Autodesk Inventor part; units mm, degrees
(part 5 of 10)
  spline S8 degree 5 poles (-8.528, -1.9637) (-8.5222, -1.9613) (-8.5144, -1.9581) (-8.5048, -1.9541) (-8.4933, -1.9493) (-8.4799, -1.9436) (-8.4704, -1.9395) (-8.461, -1.9354) (-8.4515, -1.9313) (-8.4421, -1.9272) (-8.4327, -1.9231) (-8.4234, -1.9189) (-8.4141, -1.9148) (-8.4048, -1.9106) (-8.3956, -1.9064) (-8.3864, -1.9022) (-8.3772, -1.898) (-8.3681, -1.8938) (-8.359, -1.8896) (-8.35, -1.8854) (-8.341, -1.8811) (-8.332, -1.8768) (-8.323, -1.8726) (-8.3141, -1.8683) (-8.3052, -1.864) (-8.2964, -1.8597) (-8.2876, -1.8553) (-8.2788, -1.851) (-8.2701, -1.8467) (-8.2614, -1.8423) (-8.251, -1.8371) (-8.2406, -1.8318) (-8.2303, -1.8266) (-8.2184, -1.8204) (-8.2065, -1.8142) (-8.1964, -1.8089) (-8.1864, -1.8036) (-8.1764, -1.7983) (-8.1664, -1.7929) (-8.1565, -1.7875) (-8.1467, -1.7822) (-8.1353, -1.7759) (-8.1239, -1.7696) (-8.1142, -1.7642) (-8.103, -1.7579) (-8.0919, -1.7515) (-8.0824, -1.7461) (-8.0714, -1.7397) (-8.0605, -1.7334) (-8.0512, -1.7279) (-8.0389, -1.7206) (-8.0266, -1.7133) (-8.016, -1.7069) (-8.0055, -1.7005) (-7.992, -1.6922) (-7.9817, -1.6858) (-7.9714, -1.6793) (-7.9612, -1.6729) (-7.9481, -1.6645) (-7.9381, -1.6581) (-7.9281, -1.6516) (-7.9168, -1.6442) (-7.9056, -1.6368) (-7.8973, -1.6312) (-7.8877, -1.6248) (-7.8781, -1.6183) (-7.8699, -1.6127) (-7.8605, -1.6062) (-7.8512, -1.5997) (-7.8432, -1.5942) (-7.834, -1.5877) (-7.8249, -1.5812) (-7.8171, -1.5756) (-7.8082, -1.5692) (-7.7993, -1.5627) (-7.7917, -1.5571) (-7.7829, -1.5507) (-7.7743, -1.5442) (-7.7669, -1.5387) (-7.7584, -1.5322) (-7.7499, -1.5258) (-7.7427, -1.5203) (-7.7344, -1.5138) (-7.7262, -1.5074) (-7.7192, -1.5019) (-7.7112, -1.4955) (-7.7032, -1.4891) (-7.6964, -1.4837) (-7.6885, -1.4773) (-7.6808, -1.4709) (-7.6742, -1.4655) (-7.6666, -1.4592) (-7.6591, -1.4529) (-7.6527, -1.4475) (-7.6453, -1.4412) (-7.638, -1.4349) (-7.6318, -1.4296) (-7.6247, -1.4234) (-7.6176, -1.4172) (-7.6116, -1.4119) (-7.6047, -1.4057) (-7.5979, -1.3995) (-7.5921, -1.3943) (-7.5854, -1.3882) (-7.5788, -1.3821) (-7.5732, -1.3769) (-7.5668, -1.3709) (-7.5604, -1.3649) (-7.555, -1.3598) (-7.5488, -1.3538) (-7.5427, -1.3479) (-7.5375, -1.3429) (-7.5315, -1.337) (-7.5256, -1.3312) (-7.5207, -1.3262) (-7.5149, -1.3204) (-7.5093, -1.3147) (-7.5045, -1.3098) (-7.499, -1.3041) (-7.4936, -1.2985) (-7.489, -1.2937) (-7.4837, -1.2882) (-7.4786, -1.2827) (-7.4742, -1.278) (-7.4692, -1.2725) (-7.4642, -1.2671) (-7.4601, -1.2625) (-7.4553, -1.2572) (-7.4506, -1.252) (-7.4466, -1.2475) (-7.4421, -1.2423) (-7.4376, -1.2372) (-7.4339, -1.2328) (-7.4296, -1.2278) (-7.4253, -1.2228) (-7.4218, -1.2186) (-7.4177, -1.2137) (-7.4137, -1.2089) (-7.4104, -1.2048) (-7.4065, -1.2001) (-7.4028, -1.1954) (-7.3996, -1.1915) (-7.3961, -1.1869) (-7.3925, -1.1824) (-7.3896, -1.1786) (-7.3862, -1.1743) (-7.383, -1.17) (-7.3802, -1.1664) (-7.3771, -1.1622) (-7.3741, -1.1581) (-7.3715, -1.1546) (-7.3686, -1.1507) (-7.3658, -1.1468) (-7.3635, -1.1435) (-7.3612, -1.1403) (-7.3583, -1.1361) (-7.3558, -1.1325) (-7.353, -1.1285) (-7.3504, -1.1246) (-7.3479, -1.1209) (-7.3461, -1.1181) (-7.3443, -1.1154) (-7.3429, -1.1132) (-7.3415, -1.1111) (-7.3402, -1.109) (-7.3388, -1.1069) (-7.3376, -1.1049) (-7.3364, -1.103) (-7.3352, -1.1011) (-7.334, -1.0992) (-7.3329, -1.0974) (-7.3319, -1.0957) (-7.3309, -1.094) (-7.3299, -1.0924) (-7.3289, -1.0908) (-7.328, -1.0892) (-7.3272, -1.0878) (-7.3264, -1.0864) (-7.3256, -1.085) (-7.3248, -1.0837) (-7.3241, -1.0824) (-7.3235, -1.0813) (-7.3229, -1.0801) (-7.3223, -1.0791) (-7.3217, -1.0781) (-7.3212, -1.0771) (-7.3208, -1.0763) (-7.3203, -1.0755) (-7.3199, -1.0747) (-7.3196, -1.074) (-7.3193, -1.0734) (-7.3189, -1.0728) (-7.3187, -1.0723) (-7.3186, -1.072) (-7.3185, -1.0718) (-7.3184, -1.0717) knots -1 -1 -1 -1 -1 -1 -0.9875 -0.983333 -0.979167 -0.975 -0.970833 -0.966667 -0.9625 -0.958333 -0.954167 -0.95 -0.945833 -0.941667 -0.9375 -0.933333 -0.929167 -0.925 -0.920833 -0.916667 -0.9125 -0.908333 -0.904167 -0.9 -0.895833 -0.891667 -0.8875 -0.883333 -0.879167 -0.875 -0.870833 -0.8625 -0.858333 -0.854167 -0.845833 -0.841667 -0.8375 -0.833333 -0.829167 -0.820833 -0.816667 -0.8125 -0.804167 -0.8 -0.795833 -0.7875 -0.783333 -0.779167 -0.770833 -0.766667 -0.7625 -0.75 -0.745833 -0.741667 -0.7375 -0.725 -0.720833 -0.716667 -0.7125 -0.7 -0.695833 -0.691667 -0.683333 -0.679167 -0.675 -0.666667 -0.6625 -0.658333 -0.65 -0.645833 -0.641667 -0.633333 -0.629167 -0.625 -0.616667 -0.6125 -0.608333 -0.6 -0.595833 -0.591667 -0.583333 -0.579167 -0.575 -0.566667 -0.5625 -0.558333 -0.55 -0.545833 -0.541667 -0.533333 -0.529167 -0.525 -0.516667 -0.5125 -0.508333 -0.5 -0.495833 -0.491667 -0.483333 -0.479167 -0.475 -0.466667 -0.4625 -0.458333 -0.45 -0.445833 -0.441667 -0.433333 -0.429167 -0.425 -0.416667 -0.4125 -0.408333 -0.4 -0.395833 -0.391667 -0.383333 -0.379167 -0.375 -0.366667 -0.3625 -0.358333 -0.35 -0.345833 -0.341667 -0.333333 -0.329167 -0.325 -0.316667 -0.3125 -0.308333 -0.3 -0.295833 -0.291667 -0.283333 -0.279167 -0.275 -0.266667 -0.2625 -0.258333 -0.25 -0.245833 -0.241667 -0.233333 -0.229167 -0.225 -0.216667 -0.2125 -0.208333 -0.2 -0.195833 -0.191667 -0.183333 -0.179167 -0.175 -0.170833 -0.158333 -0.154167 -0.145833 -0.141667 -0.1375 -0.133333 -0.129167 -0.125 -0.120833 -0.116667 -0.1125 -0.108333 -0.104167 -0.1 -0.095833 -0.091667 -0.0875 -0.083333 -0.079167 -0.075 -0.070833 -0.066667 -0.0625 -0.058333 -0.054167 -0.05 -0.045833 -0.041667 -0.0375 -0.033333 -0.029167 -0.025 -0.020833 -0.016667 -0.0125 -0.008333 0 0 0 0 0 0
  line L18 (-0.374, 5.4756) -> (0.4714, 5.7477)
  line L19 (0.4714, 5.7477) -> (0.472, 5.7479)
  spline S9 degree 5 poles (0.472, 5.7479) (0.4721, 5.7479) (0.4722, 5.748) (0.4724, 5.7481) (0.4728, 5.7482) (0.4733, 5.7483) (0.4738, 5.7485) (0.4745, 5.7488) (0.4752, 5.749) (0.476, 5.7493) (0.4768, 5.7496) (0.4778, 5.75) (0.4788, 5.7504) (0.4798, 5.7508) (0.4809, 5.7512) (0.4821, 5.7517) (0.4834, 5.7522) (0.4847, 5.7527) (0.4861, 5.7533) (0.4876, 5.7539) (0.4891, 5.7545) (0.4907, 5.7551) (0.4923, 5.7558) (0.494, 5.7566) (0.4957, 5.7573) (0.4976, 5.7581) (0.4994, 5.7589) (0.5014, 5.7598) (0.5033, 5.7607) (0.5054, 5.7616) (0.5075, 5.7625) (0.5096, 5.7635) (0.5123, 5.7647) (0.515, 5.766) (0.5178, 5.7674) (0.5212, 5.769) (0.5246, 5.7707) (0.5277, 5.7722) (0.5313, 5.774) (0.535, 5.7758) (0.5383, 5.7775) (0.5422, 5.7795) (0.5462, 5.7816) (0.5497, 5.7834) (0.5539, 5.7856) (0.5581, 5.7879) (0.5618, 5.79) (0.5662, 5.7924) (0.5707, 5.7949) (0.5746, 5.797) (0.5793, 5.7997) (0.584, 5.8024) (0.5881, 5.8047) (0.5929, 5.8076) (0.5979, 5.8105) (0.6022, 5.813) (0.6072, 5.8161) (0.6124, 5.8192) (0.6168, 5.8219) (0.6221, 5.8252) (0.6274, 5.8285) (0.632, 5.8314) (0.6375, 5.8349) (0.643, 5.8385) (0.6478, 5.8416) (0.6534, 5.8453) (0.6591, 5.849) (0.664, 5.8523) (0.6698, 5.8562) (0.6757, 5.8602) (0.6807, 5.8637) (0.6867, 5.8678) (0.6927, 5.872) (0.6979, 5.8757) (0.704, 5.88) (0.7102, 5.8844) (0.7155, 5.8883) (0.7218, 5.8929) (0.7281, 5.8975) (0.7335, 5.9015) (0.7399, 5.9063) (0.7464, 5.9112) (0.7519, 5.9154) (0.7585, 5.9204) (0.765, 5.9255) (0.7707, 5.93) (0.7774, 5.9352) (0.784, 5.9405) (0.7898, 5.9451) (0.7966, 5.9506) (0.8034, 5.9561) (0.8092, 5.9609) (0.8161, 5.9666) (0.823, 5.9723) (0.829, 5.9773) (0.8359, 5.9832) (0.8429, 5.9892) (0.849, 5.9944) (0.856, 6.0005) (0.8631, 6.0067) (0.8692, 6.0121) (0.8764, 6.0185) (0.8836, 6.0249) (0.8897, 6.0305) (0.897, 6.037) (0.9042, 6.0437) (0.9105, 6.0494) (0.9178, 6.0562) (0.9251, 6.0631) (0.9314, 6.0691) (0.9388, 6.0761) (0.9462, 6.0832) (0.9525, 6.0893) (0.96, 6.0966) (0.9674, 6.1039) (0.9738, 6.1102) (0.9813, 6.1177) (0.9888, 6.1252) (0.9953, 6.1318) (1.0028, 6.1395) (1.0104, 6.1472) (1.0169, 6.1539) (1.0244, 6.1618) (1.032, 6.1698) (1.0386, 6.1767) (1.0462, 6.1849) (1.0538, 6.1931) (1.0604, 6.2002) (1.0681, 6.2085) (1.0757, 6.217) (1.0823, 6.2243) (1.09, 6.2328) (1.0977, 6.2415) (1.1043, 6.249) (1.112, 6.2577) (1.1197, 6.2666) (1.1264, 6.2743) (1.1341, 6.2833) (1.1418, 6.2924) (1.1485, 6.3002) (1.1562, 6.3095) (1.164, 6.3188) (1.1706, 6.3268) (1.1784, 6.3362) (1.1861, 6.3458) (1.1928, 6.354) (1.2005, 6.3637) (1.2083, 6.3734) (1.215, 6.3818) (1.2216, 6.3903) (1.2316, 6.4031) (1.2404, 6.4145) (1.2493, 6.4261) (1.2582, 6.4378) (1.2692, 6.4525) (1.277, 6.4629) (1.2847, 6.4734) (1.2924, 6.484) (1.3035, 6.4992) (1.3123, 6.5114) (1.3211, 6.5238) (1.3299, 6.5362) (1.3387, 6.5488) (1.3442, 6.5567) (1.3496, 6.5647) (1.3551, 6.5726) (1.3606, 6.5806) (1.3661, 6.5887) (1.3715, 6.5968) (1.377, 6.6049) (1.3824, 6.613) (1.3879, 6.6212) (1.3933, 6.6295) (1.3987, 6.6377) (1.4041, 6.646) (1.4096, 6.6544) (1.415, 6.6628) (1.4204, 6.6712) (1.4258, 6.6796) (1.4312, 6.6881) (1.4365, 6.6966) (1.4419, 6.7052) (1.4473, 6.7138) (1.4526, 6.7224) (1.458, 6.7311) (1.4633, 6.7398) (1.4687, 6.7486) (1.474, 6.7573) (1.4793, 6.7662) (1.4846, 6.775) (1.4899, 6.7839) (1.4973, 6.7964) (1.5036, 6.8071) (1.5089, 6.8162) (1.5131, 6.8234) (1.5162, 6.8289) knots 0 0 0 0 0 0 0.004167 0.008333 0.0125 0.016667 0.020833 0.025 0.029167 0.033333 0.0375 0.041667 0.045833 0.05 0.054167 0.058333 0.0625 0.066667 0.070833 0.075 0.079167 0.083333 0.0875 0.091667 0.095833 0.1 0.104167 0.108333 0.1125 0.116667 0.120833 0.125 0.129167 0.1375 0.141667 0.145833 0.154167 0.158333 0.1625 0.170833 0.175 0.179167 0.1875 0.191667 0.195833 0.204167 0.208333 0.2125 0.220833 0.225 0.229167 0.2375 0.241667 0.245833 0.254167 0.258333 0.2625 0.270833 0.275 0.279167 0.2875 0.291667 0.295833 0.304167 0.308333 0.3125 0.320833 0.325 0.329167 0.3375 0.341667 0.345833 0.354167 0.358333 0.3625 0.370833 0.375 0.379167 0.3875 0.391667 0.395833 0.404167 0.408333 0.4125 0.420833 0.425 0.429167 0.4375 0.441667 0.445833 0.454167 0.458333 0.4625 0.470833 0.475 0.479167 0.4875 0.491667 0.495833 0.504167 0.508333 0.5125 0.520833 0.525 0.529167 0.5375 0.541667 0.545833 0.554167 0.558333 0.5625 0.570833 0.575 0.579167 0.5875 0.591667 0.595833 0.604167 0.608333 0.6125 0.620833 0.625 0.629167 0.6375 0.641667 0.645833 0.654167 0.658333 0.6625 0.670833 0.675 0.679167 0.6875 0.691667 0.695833 0.704167 0.708333 0.7125 0.720833 0.725 0.729167 0.7375 0.741667 0.745833 0.754167 0.758333 0.7625 0.770833 0.775 0.779167 0.783333 0.8 0.804167 0.808333 0.8125 0.825 0.829167 0.833333 0.8375 0.854167 0.858333 0.8625 0.866667 0.870833 0.875 0.879167 0.883333 0.8875 0.891667 0.895833 0.9 0.904167 0.908333 0.9125 0.916667 0.920833 0.925 0.929167 0.933333 0.9375 0.941667 0.945833 0.95 0.954167 0.958333 0.9625 0.966667 0.970833 0.975 0.979167 0.983333 0.9875 1 1 1 1 1 1
  arc A10 (1.5162, 6.8289) -> (1.2422, 7.3858) centre (-4.8955, 4.02) ccw
  spline S10 degree 5 poles (1.2422, 7.3858) (1.236, 7.3866) (1.2277, 7.3877) (1.2173, 7.3891) (1.2049, 7.3906) (1.1905, 7.3924) (1.1802, 7.3936) (1.17, 7.3948) (1.1598, 7.396) (1.1496, 7.3971) (1.1394, 7.3982) (1.1292, 7.3993) (1.1191, 7.4003) (1.109, 7.4014) (1.0989, 7.4024) (1.0888, 7.4033) (1.0788, 7.4043) (1.0688, 7.4052) (1.0588, 7.4061) (1.0488, 7.4069) (1.0389, 7.4077) (1.029, 7.4085) (1.0191, 7.4093) (1.0092, 7.4101) (0.9994, 7.4108) (0.9896, 7.4115) (0.9798, 7.4121) (0.97, 7.4128) (0.9603, 7.4134) (0.9506, 7.4139) (0.939, 7.4146) (0.9274, 7.4152) (0.9158, 7.4158) (0.9024, 7.4164) (0.8891, 7.417) (0.8776, 7.4175) (0.8663, 7.4179) (0.8549, 7.4183) (0.8436, 7.4186) (0.8324, 7.4189) (0.8212, 7.4192) (0.8082, 7.4195) (0.7952, 7.4197) (0.7841, 7.4199) (0.7712, 7.42) (0.7584, 7.4201) (0.7475, 7.4201) (0.7348, 7.4201) (0.7221, 7.42) (0.7114, 7.42) (0.697, 7.4198) (0.6828, 7.4196) (0.6704, 7.4193) (0.658, 7.419) (0.6423, 7.4186) (0.6301, 7.4182) (0.6179, 7.4178) (0.6059, 7.4173) (0.5904, 7.4166) (0.5785, 7.416) (0.5666, 7.4154) (0.5548, 7.4147) (0.5397, 7.4138) (0.5281, 7.4131) (0.5165, 7.4123) (0.5033, 7.4113) (0.4903, 7.4103) (0.4805, 7.4095) (0.4692, 7.4085) (0.458, 7.4075) (0.4484, 7.4067) (0.4373, 7.4056) (0.4262, 7.4045) (0.4168, 7.4035) (0.4059, 7.4023) (0.395, 7.4011) (0.3858, 7.4001) (0.3751, 7.3988) (0.3645, 7.3975) (0.3554, 7.3963) (0.3449, 7.395) (0.3344, 7.3936) (0.3256, 7.3923) (0.3153, 7.3909) (0.305, 7.3894) (0.2963, 7.3881) (0.2863, 7.3865) (0.2763, 7.3849) (0.2677, 7.3836) (0.2579, 7.3819) (0.2481, 7.3803) (0.2398, 7.3788) (0.2301, 7.3771) (0.2206, 7.3754) (0.2124, 7.3739) (0.203, 7.3721) (0.1937, 7.3703) (0.1857, 7.3687) (0.1765, 7.3669) (0.1674, 7.365) (0.1597, 7.3634) (0.1507, 7.3614) (0.1419, 7.3595) (0.1343, 7.3578) (0.1256, 7.3559) (0.117, 7.3539) (0.1097, 7.3521) (0.1012, 7.3501) (0.0928, 7.3481) (0.0857, 7.3463) (0.0775, 7.3442) (0.0693, 7.3422) (0.0624, 7.3404) (0.0544, 7.3382) (0.0465, 7.3361) (0.0399, 7.3343) (0.0321, 7.3321) (0.0245, 7.33) (0.018, 7.3281) (0.0106, 7.326) (0.0032, 7.3238) (-0.003, 7.3219) (-0.0103, 7.3197) (-0.0174, 7.3175) (-0.0234, 7.3156) (-0.0303, 7.3134) (-0.0372, 7.3112) (-0.0429, 7.3093) (-0.0496, 7.3071) (-0.0562, 7.3049) (-0.0617, 7.303) (-0.0681, 7.3008) (-0.0744, 7.2986) (-0.0797, 7.2967) (-0.0858, 7.2945) (-0.0918, 7.2923) (-0.0969, 7.2904) (-0.1027, 7.2883) (-0.1084, 7.2861) (-0.1133, 7.2842) (-0.1188, 7.2821) (-0.1242, 7.2799) (-0.1288, 7.2781) (-0.134, 7.276) (-0.1392, 7.2739) (-0.1435, 7.2721) (-0.1484, 7.27) (-0.1532, 7.2679) (-0.1573, 7.2662) (-0.1619, 7.2642) (-0.1665, 7.2622) (-0.1702, 7.2605) (-0.1746, 7.2585) (-0.1788, 7.2566) (-0.1823, 7.255) (-0.1863, 7.2531) (-0.1902, 7.2512) (-0.1935, 7.2497) (-0.1972, 7.2479) (-0.2007, 7.2461) (-0.2037, 7.2447) (-0.2066, 7.2432) (-0.2094, 7.2418) (-0.2117, 7.2406) (-0.2139, 7.2395) (-0.216, 7.2384) (-0.2181, 7.2373) (-0.2202, 7.2362) (-0.2221, 7.2351) (-0.2241, 7.2341) (-0.2259, 7.2331) (-0.2277, 7.2321) (-0.2294, 7.2311) (-0.2311, 7.2302) (-0.2327, 7.2293) (-0.2342, 7.2284) (-0.2357, 7.2276) (-0.2371, 7.2268) (-0.2385, 7.226) (-0.2398, 7.2252) (-0.241, 7.2245) (-0.2422, 7.2238) (-0.2433, 7.2231) (-0.2443, 7.2225) (-0.2453, 7.2219) (-0.2462, 7.2214) (-0.247, 7.2208) (-0.2478, 7.2204) (-0.2485, 7.2199) (-0.2492, 7.2195) (-0.2497, 7.2191) (-0.2503, 7.2187) (-0.2508, 7.2185) (-0.2511, 7.2183) (-0.2512, 7.2182) (-0.2513, 7.2181) knots -1 -1 -1 -1 -1 -1 -0.9875 -0.983333 -0.979167 -0.975 -0.970833 -0.966667 -0.9625 -0.958333 -0.954167 -0.95 -0.945833 -0.941667 -0.9375 -0.933333 -0.929167 -0.925 -0.920833 -0.916667 -0.9125 -0.908333 -0.904167 -0.9 -0.895833 -0.891667 -0.8875 -0.883333 -0.879167 -0.875 -0.870833 -0.8625 -0.858333 -0.854167 -0.845833 -0.841667 -0.8375 -0.833333 -0.829167 -0.820833 -0.816667 -0.8125 -0.804167 -0.8 -0.795833 -0.7875 -0.783333 -0.779167 -0.770833 -0.766667 -0.7625 -0.75 -0.745833 -0.741667 -0.7375 -0.725 -0.720833 -0.716667 -0.7125 -0.7 -0.695833 -0.691667 -0.6875 -0.675 -0.670833 -0.666667 -0.658333 -0.654167 -0.65 -0.641667 -0.6375 -0.633333 -0.625 -0.620833 -0.616667 -0.608333 -0.604167 -0.6 -0.591667 -0.5875 -0.583333 -0.575 -0.570833 -0.566667 -0.558333 -0.554167 -0.55 -0.541667 -0.5375 -0.533333 -0.525 -0.520833 -0.516667 -0.508333 -0.504167 -0.5 -0.491667 -0.4875 -0.483333 -0.475 -0.470833 -0.466667 -0.458333 -0.454167 -0.45 -0.441667 -0.4375 -0.433333 -0.425 -0.420833 -0.416667 -0.408333 -0.404167 -0.4 -0.391667 -0.3875 -0.383333 -0.375 -0.370833 -0.366667 -0.358333 -0.354167 -0.35 -0.341667 -0.3375 -0.333333 -0.325 -0.320833 -0.316667 -0.308333 -0.304167 -0.3 -0.291667 -0.2875 -0.283333 -0.275 -0.270833 -0.266667 -0.258333 -0.254167 -0.25 -0.241667 -0.2375 -0.233333 -0.225 -0.220833 -0.216667 -0.208333 -0.204167 -0.2 -0.191667 -0.1875 -0.183333 -0.175 -0.170833 -0.166667 -0.158333 -0.154167 -0.15 -0.141667 -0.1375 -0.133333 -0.129167 -0.125 -0.120833 -0.116667 -0.1125 -0.108333 -0.104167 -0.1 -0.095833 -0.091667 -0.0875 -0.083333 -0.079167 -0.075 -0.070833 -0.066667 -0.0625 -0.058333 -0.054167 -0.05 -0.045833 -0.041667 -0.0375 -0.033333 -0.029167 -0.025 -0.020833 -0.016667 -0.0125 -0.008333 0 0 0 0 0 0
  line L20 (-0.2519, 7.2177) -> (-0.9834, 6.714)
  line L21 (-0.2513, 7.2181) -> (-0.2519, 7.2177)
  arc A11 (-0.9834, 6.714) -> (-1.7076, 7.5413) centre (-4.8955, 4.02) ccw
  line L22 (-1.7076, 7.5413) -> (-1.1115, 8.1997)
  line L23 (-2.4726, 9.1117) -> (-2.4729, 9.1111)
  line L24 (-2.4729, 9.1111) -> (-2.8545, 8.3091)
  spline S11 degree 5 poles (-1.1111, 8.2002) (-1.111, 8.2002) (-1.1109, 8.2003) (-1.1108, 8.2005) (-1.1105, 8.2008) (-1.1102, 8.2012) (-1.1098, 8.2016) (-1.1094, 8.2022) (-1.1089, 8.2027) (-1.1083, 8.2034) (-1.1078, 8.2041) (-1.1071, 8.2048) (-1.1065, 8.2057) (-1.1057, 8.2066) (-1.105, 8.2075) (-1.1042, 8.2085) (-1.1033, 8.2096) (-1.1024, 8.2107) (-1.1015, 8.2119) (-1.1006, 8.2131) (-1.0996, 8.2144) (-1.0985, 8.2158) (-1.0975, 8.2172) (-1.0964, 8.2186) (-1.0952, 8.2202) (-1.094, 8.2218) (-1.0928, 8.2234) (-1.0916, 8.2251) (-1.0903, 8.2269) (-1.089, 8.2287) (-1.0877, 8.2306) (-1.0863, 8.2325) (-1.0846, 8.2349) (-1.0829, 8.2373) (-1.0811, 8.2399) (-1.079, 8.243) (-1.0769, 8.2462) (-1.075, 8.249) (-1.0727, 8.2524) (-1.0704, 8.2559) (-1.0684, 8.259) (-1.0664, 8.2621) (-1.064, 8.2659) (-1.0608, 8.2709) (-1.0576, 8.2761) (-1.0543, 8.2815) (-1.0509, 8.287) (-1.0475, 8.2928) (-1.0448, 8.2973) (-1.0421, 8.302) (-1.0393, 8.3067) (-1.0362, 8.3123) (-1.0333, 8.3173) (-1.0309, 8.3216) (-1.0281, 8.3268) (-1.0252, 8.3321) (-1.0227, 8.3367) (-1.0198, 8.3421) (-1.0168, 8.3477) (-1.0143, 8.3525) (-1.0113, 8.3582) (-1.0083, 8.3641) (-1.0057, 8.3692) (-1.0027, 8.3752) (-0.9996, 8.3813) (-0.997, 8.3866) (-0.9939, 8.3929) (-0.9908, 8.3992) (-0.9882, 8.4048) (-0.9851, 8.4113) (-0.982, 8.418) (-0.9793, 8.4238) (-0.9762, 8.4306) (-0.9731, 8.4375) (-0.9704, 8.4435) (-0.9672, 8.4506) (-0.9641, 8.4578) (-0.9614, 8.464) (-0.9582, 8.4713) (-0.9551, 8.4788) (-0.9524, 8.4852) (-0.9492, 8.4928) (-0.9461, 8.5005) (-0.9434, 8.5072) (-0.9403, 8.515) (-0.9371, 8.523) (-0.9344, 8.5298) (-0.9313, 8.5379) (-0.9282, 8.5461) (-0.9255, 8.5532) (-0.9224, 8.5616) (-0.9193, 8.57) (-0.9166, 8.5773) (-0.9136, 8.5859) (-0.9105, 8.5946) (-0.9079, 8.6021) (-0.9048, 8.6109) (-0.9018, 8.6199) (-0.8992, 8.6276) (-0.8961, 8.6366) (-0.8931, 8.6458) (-0.8906, 8.6537) (-0.8876, 8.663) (-0.8846, 8.6724) (-0.8821, 8.6805) (-0.8792, 8.6901) (-0.8763, 8.6997) (-0.8738, 8.708) (-0.8709, 8.7178) (-0.8681, 8.7276) (-0.8656, 8.7361) (-0.8628, 8.7461) (-0.86, 8.7562) (-0.8576, 8.7649) (-0.8549, 8.7751) (-0.8522, 8.7854) (-0.8498, 8.7942) (-0.8471, 8.8047) (-0.8445, 8.8152) (-0.8422, 8.8242) (-0.8396, 8.8349) (-0.837, 8.8456) (-0.8348, 8.8548) (-0.8323, 8.8657) (-0.8298, 8.8766) (-0.8276, 8.886) (-0.8252, 8.8971) (-0.8228, 8.9082) (-0.8207, 8.9178) (-0.8183, 8.9291) (-0.816, 8.9405) (-0.814, 8.9502) (-0.8117, 8.9617) (-0.8095, 8.9732) (-0.8076, 8.9832) (-0.8054, 8.9949) (-0.8032, 9.0066) (-0.8014, 9.0167) (-0.7993, 9.0286) (-0.7972, 9.0405) (-0.7955, 9.0508) (-0.7935, 9.0629) (-0.7915, 9.075) (-0.7899, 9.0854) (-0.788, 9.0977) (-0.7862, 9.11) (-0.7846, 9.1206) (-0.7826, 9.1348) (-0.7806, 9.1491) (-0.7789, 9.1617) (-0.7772, 9.1743) (-0.7756, 9.1871) (-0.7738, 9.2017) (-0.7721, 9.2163) (-0.7704, 9.2311) (-0.7688, 9.2459) (-0.767, 9.2628) (-0.7659, 9.274) (-0.7648, 9.2853) (-0.7633, 9.3004) (-0.762, 9.3156) (-0.7608, 9.329) (-0.7597, 9.3424) (-0.7586, 9.3559) (-0.7579, 9.3656) (-0.7572, 9.3753) (-0.7565, 9.3851) (-0.7558, 9.3948) (-0.7552, 9.4046) (-0.7546, 9.4144) (-0.754, 9.4243) (-0.7534, 9.4341) (-0.7529, 9.444) (-0.7524, 9.454) (-0.7519, 9.4639) (-0.7514, 9.4739) (-0.7509, 9.4839) (-0.7505, 9.494) (-0.7501, 9.5041) (-0.7498, 9.5142) (-0.7494, 9.5243) (-0.7491, 9.5344) (-0.7488, 9.5446) (-0.7485, 9.5548) (-0.7483, 9.5651) (-0.748, 9.5753) (-0.7479, 9.5856) (-0.7477, 9.5959) (-0.7475, 9.6063) (-0.7474, 9.6208) (-0.7473, 9.6333) (-0.7472, 9.6437) (-0.7472, 9.6521) (-0.7472, 9.6584) knots 0 0 0 0 0 0 0.004167 0.008333 0.0125 0.016667 0.020833 0.025 0.029167 0.033333 0.0375 0.041667 0.045833 0.05 0.054167 0.058333 0.0625 0.066667 0.070833 0.075 0.079167 0.083333 0.0875 0.091667 0.095833 0.1 0.104167 0.108333 0.1125 0.116667 0.120833 0.125 0.129167 0.1375 0.141667 0.145833 0.154167 0.158333 0.1625 0.170833 0.175 0.179167 0.183333 0.191667 0.208333 0.2125 0.216667 0.220833 0.229167 0.2375 0.241667 0.245833 0.254167 0.258333 0.2625 0.270833 0.275 0.279167 0.2875 0.291667 0.295833 0.304167 0.308333 0.3125 0.320833 0.325 0.329167 0.3375 0.341667 0.345833 0.354167 0.358333 0.3625 0.370833 0.375 0.379167 0.3875 0.391667 0.395833 0.404167 0.408333 0.4125 0.420833 0.425 0.429167 0.4375 0.441667 0.445833 0.454167 0.458333 0.4625 0.470833 0.475 0.479167 0.4875 0.491667 0.495833 0.504167 0.508333 0.5125 0.520833 0.525 0.529167 0.5375 0.541667 0.545833 0.554167 0.558333 0.5625 0.570833 0.575 0.579167 0.5875 0.591667 0.595833 0.604167 0.608333 0.6125 0.620833 0.625 0.629167 0.6375 0.641667 0.645833 0.654167 0.658333 0.6625 0.670833 0.675 0.679167 0.6875 0.691667 0.695833 0.704167 0.708333 0.7125 0.720833 0.725 0.729167 0.7375 0.741667 0.745833 0.754167 0.758333 0.7625 0.770833 0.775 0.779167 0.791667 0.795833 0.8 0.804167 0.808333 0.825 0.829167 0.833333 0.8375 0.845833 0.85 0.854167 0.866667 0.870833 0.875 0.879167 0.883333 0.8875 0.891667 0.895833 0.9 0.904167 0.908333 0.9125 0.916667 0.920833 0.925 0.929167 0.933333 0.9375 0.941667 0.945833 0.95 0.954167 0.958333 0.9625 0.966667 0.970833 0.975 0.979167 0.983333 0.9875 1 1 1 1 1 1
  arc A12 (-0.7472, 9.6584) -> (-1.263, 10.0037) centre (-4.8955, 4.02) ccw
  spline S12 degree 5 poles (-1.263, 10.0037) (-1.2688, 10.0013) (-1.2766, 9.9981) (-1.2862, 9.9941) (-1.2977, 9.9892) (-1.3111, 9.9836) (-1.3206, 9.9795) (-1.33, 9.9754) (-1.3395, 9.9713) (-1.3489, 9.9672) (-1.3583, 9.963) (-1.3676, 9.9589) (-1.3769, 9.9548) (-1.3862, 9.9506) (-1.3954, 9.9464) (-1.4046, 9.9422) (-1.4138, 9.938) (-1.4229, 9.9338) (-1.432, 9.9296) (-1.441, 9.9253) (-1.45, 9.9211) (-1.459, 9.9168) (-1.468, 9.9125) (-1.4769, 9.9082) (-1.4858, 9.9039) (-1.4946, 9.8996) (-1.5034, 9.8953) (-1.5122, 9.891) (-1.5209, 9.8866) (-1.5296, 9.8823) (-1.54, 9.877) (-1.5504, 9.8718) (-1.5607, 9.8665) (-1.5726, 9.8604) (-1.5844, 9.8542) (-1.5946, 9.8489) (-1.6046, 9.8436) (-1.6146, 9.8382) (-1.6246, 9.8329) (-1.6345, 9.8275) (-1.6443, 9.8221) (-1.6557, 9.8159) (-1.6671, 9.8096) (-1.6768, 9.8042) (-1.688, 9.7978) (-1.6991, 9.7915) (-1.7086, 9.7861) (-1.7196, 9.7797) (-1.7305, 9.7733) (-1.7398, 9.7679) (-1.7521, 9.7606) (-1.7644, 9.7533) (-1.775, 9.7468) (-1.7855, 9.7404) (-1.799, 9.7322) (-1.8093, 9.7257) (-1.8196, 9.7193) (-1.8298, 9.7128) (-1.8429, 9.7045) (-1.8529, 9.698) (-1.8629, 9.6916) (-1.8742, 9.6842) (-1.8854, 9.6768) (-1.8937, 9.6712) (-1.9033, 9.6647) (-1.9129, 9.6582) (-1.9211, 9.6527) (-1.9305, 9.6462) (-1.9398, 9.6397) (-1.9478, 9.6341) (-1.957, 9.6277) (-1.9661, 9.6212) (-1.9739, 9.6156) (-1.9828, 9.6091) (-1.9917, 9.6027) (-1.9993, 9.5971) (-2.0081, 9.5906) (-2.0167, 9.5842) (-2.0241, 9.5786) (-2.0326, 9.5722) (-2.0411, 9.5657) (-2.0483, 9.5602) (-2.0566, 9.5538) (-2.0648, 9.5474) (-2.0718, 9.5419) (-2.0798, 9.5355) (-2.0878, 9.5291) (-2.0946, 9.5236) (-2.1025, 9.5173) (-2.1102, 9.5109) (-2.1168, 9.5055) (-2.1244, 9.4992) (-2.1319, 9.4928) (-2.1383, 9.4875) (-2.1457, 9.4812) (-2.153, 9.4749) (-2.1592, 9.4696) (-2.1663, 9.4633) (-2.1734, 9.4571) (-2.1794, 9.4518) (-2.1863, 9.4457) (-2.1931, 9.4395) (-2.1989, 9.4343) (-2.2056, 9.4282) (-2.2122, 9.4221) (-2.2178, 9.4169) (-2.2242, 9.4109) (-2.2306, 9.4049) (-2.236, 9.3998) (-2.2422, 9.3938) (-2.2483, 9.3879) (-2.2535, 9.3828) (-2.2595, 9.377) (-2.2654, 9.3711) (-2.2703, 9.3662) (-2.2761, 9.3604) (-2.2817, 9.3547) (-2.2865, 9.3498) (-2.292, 9.3441) (-2.2974, 9.3385) (-2.302, 9.3337) (-2.3073, 9.3281) (-2.3124, 9.3226) (-2.3168, 9.3179) (-2.3218, 9.3125) (-2.3268, 9.3071) (-2.3309, 9.3025) (-2.3357, 9.2972) (-2.3404, 9.2919) (-2.3444, 9.2874) (-2.3489, 9.2823) (-2.3534, 9.2771) (-2.3571, 9.2728) (-2.3614, 9.2677) (-2.3657, 9.2628) (-2.3692, 9.2585) (-2.3733, 9.2537) (-2.3773, 9.2488) (-2.3806, 9.2447) (-2.3845, 9.24) (-2.3882, 9.2354) (-2.3913, 9.2314) (-2.3949, 9.2269) (-2.3985, 9.2224) (-2.4014, 9.2186) (-2.4048, 9.2142) (-2.408, 9.2099) (-2.4108, 9.2063) (-2.4139, 9.2021) (-2.4169, 9.1981) (-2.4195, 9.1946) (-2.4224, 9.1906) (-2.4252, 9.1868) (-2.4275, 9.1835) (-2.4298, 9.1803) (-2.4327, 9.1761) (-2.4352, 9.1725) (-2.438, 9.1685) (-2.4406, 9.1646) (-2.4431, 9.1608) (-2.4449, 9.1581) (-2.4467, 9.1554) (-2.4481, 9.1532) (-2.4495, 9.1511) (-2.4508, 9.149) (-2.4522, 9.1469) (-2.4534, 9.1449) (-2.4546, 9.143) (-2.4558, 9.1411) (-2.457, 9.1392) (-2.4581, 9.1374) (-2.4591, 9.1357) (-2.4601, 9.134) (-2.4611, 9.1323) (-2.4621, 9.1307) (-2.463, 9.1292) (-2.4638, 9.1277) (-2.4646, 9.1263) (-2.4654, 9.125) (-2.4662, 9.1237) (-2.4669, 9.1224) (-2.4675, 9.1212) (-2.4681, 9.1201) (-2.4687, 9.119) (-2.4693, 9.118) (-2.4698, 9.1171) (-2.4702, 9.1162) (-2.4707, 9.1154) (-2.4711, 9.1147) (-2.4714, 9.114) (-2.4717, 9.1134) (-2.4721, 9.1128) (-2.4723, 9.1123) (-2.4724, 9.112) (-2.4725, 9.1118) (-2.4726, 9.1117) knots -1 -1 -1 -1 -1 -1 -0.9875 -0.983333 -0.979167 -0.975 -0.970833 -0.966667 -0.9625 -0.958333 -0.954167 -0.95 -0.945833 -0.941667 -0.9375 -0.933333 -0.929167 -0.925 -0.920833 -0.916667 -0.9125 -0.908333 -0.904167 -0.9 -0.895833 -0.891667 -0.8875 -0.883333 -0.879167 -0.875 -0.870833 -0.8625 -0.858333 -0.854167 -0.845833 -0.841667 -0.8375 -0.833333 -0.829167 -0.820833 -0.816667 -0.8125 -0.804167 -0.8 -0.795833 -0.7875 -0.783333 -0.779167 -0.770833 -0.766667 -0.7625 -0.75 -0.745833 -0.741667 -0.7375 -0.725 -0.720833 -0.716667 -0.7125 -0.7 -0.695833 -0.691667 -0.683333 -0.679167 -0.675 -0.666667 -0.6625 -0.658333 -0.65 -0.645833 -0.641667 -0.633333 -0.629167 -0.625 -0.616667 -0.6125 -0.608333 -0.6 -0.595833 -0.591667 -0.583333 -0.579167 -0.575 -0.566667 -0.5625 -0.558333 -0.55 -0.545833 -0.541667 -0.533333 -0.529167 -0.525 -0.516667 -0.5125 -0.508333 -0.5 -0.495833 -0.491667 -0.483333 -0.479167 -0.475 -0.466667 -0.4625 -0.458333 -0.45 -0.445833 -0.441667 -0.433333 -0.429167 -0.425 -0.416667 -0.4125 -0.408333 -0.4 -0.395833 -0.391667 -0.383333 -0.379167 -0.375 -0.366667 -0.3625 -0.358333 -0.35 -0.345833 -0.341667 -0.333333 -0.329167 -0.325 -0.316667 -0.3125 -0.308333 -0.3 -0.295833 -0.291667 -0.283333 -0.279167 -0.275 -0.266667 -0.2625 -0.258333 -0.25 -0.245833 -0.241667 -0.233333 -0.229167 -0.225 -0.216667 -0.2125 -0.208333 -0.2 -0.195833 -0.191667 -0.183333 -0.179167 -0.175 -0.170833 -0.158333 -0.154167 -0.145833 -0.141667 -0.1375 -0.133333 -0.129167 -0.125 -0.120833 -0.116667 -0.1125 -0.108333 -0.104167 -0.1 -0.095833 -0.091667 -0.0875 -0.083333 -0.079167 -0.075 -0.070833 -0.066667 -0.0625 -0.058333 -0.054167 -0.05 -0.045833 -0.041667 -0.0375 -0.033333 -0.029167 -0.025 -0.020833 -0.016667 -0.0125 -0.008333 0 0 0 0 0 0
  line L25 (-1.1115, 8.1997) -> (-1.1111, 8.2002)
  arc A13 (-2.8545, 8.3091) -> (-3.8953, 8.6635) centre (-4.8955, 4.02) ccw
  line L26 (-3.7083, 9.5317) -> (-3.7082, 9.5324)
  line L27 (-3.8953, 8.6635) -> (-3.7083, 9.5317)
  spline S13 degree 5 poles (-3.7082, 9.5324) (-3.7082, 9.5324) (-3.7081, 9.5326) (-3.7081, 9.5328) (-3.708, 9.5331) (-3.7079, 9.5336) (-3.7078, 9.5342) (-3.7077, 9.5349) (-3.7076, 9.5357) (-3.7074, 9.5365) (-3.7073, 9.5374) (-3.7071, 9.5384) (-3.7069, 9.5394) (-3.7068, 9.5405) (-3.7066, 9.5417) (-3.7064, 9.543) (-3.7062, 9.5443) (-3.706, 9.5458) (-3.7058, 9.5472) (-3.7056, 9.5488) (-3.7053, 9.5504) (-3.7051, 9.5521) (-3.7049, 9.5539) (-3.7047, 9.5557) (-3.7044, 9.5576) (-3.7042, 9.5596) (-3.704, 9.5616) (-3.7038, 9.5637) (-3.7035, 9.5659) (-3.7033, 9.5681) (-3.7031, 9.5704) (-3.7029, 9.5727) (-3.7026, 9.5756) (-3.7024, 9.5786) (-3.7021, 9.5817) (-3.7018, 9.5854) (-3.7016, 9.5893) (-3.7013, 9.5927) (-3.7011, 9.5967) (-3.7008, 9.6009) (-3.7006, 9.6046) (-3.7004, 9.609) (-3.7002, 9.6135) (-3.7001, 9.6174) (-3.6999, 9.6221) (-3.6998, 9.6269) (-3.6997, 9.6312) (-3.6996, 9.6362) (-3.6995, 9.6413) (-3.6994, 9.6458) (-3.6994, 9.6511) (-3.6993, 9.6566) (-3.6994, 9.6613) (-3.6994, 9.6669) (-3.6994, 9.6726) (-3.6995, 9.6776) (-3.6996, 9.6835) (-3.6997, 9.6895) (-3.6999, 9.6948) (-3.7001, 9.7009) (-3.7003, 9.7072) (-3.7005, 9.7127) (-3.7008, 9.7191) (-3.7011, 9.7257) (-3.7014, 9.7314) (-3.7018, 9.7381) (-3.7022, 9.7449) (-3.7026, 9.7508) (-3.7031, 9.7578) (-3.7036, 9.7649) (-3.7041, 9.771) (-3.7047, 9.7782) (-3.7053, 9.7855) (-3.7059, 9.7919) (-3.7066, 9.7993) (-3.7073, 9.8069) (-3.708, 9.8134) (-3.7088, 9.8211) (-3.7097, 9.8289) (-3.7105, 9.8357) (-3.7114, 9.8436) (-3.7124, 9.8516) (-3.7133, 9.8585) (-3.7144, 9.8667) (-3.7155, 9.8749) (-3.7165, 9.882) (-3.7177, 9.8904) (-3.7189, 9.8989) (-3.7201, 9.9062) (-3.7214, 9.9147) (-3.7228, 9.9234) (-3.724, 9.9309) (-3.7255, 9.9397) (-3.727, 9.9485) (-3.7284, 9.9562) (-3.73, 9.9652) (-3.7317, 9.9742) (-3.7332, 9.982) (-3.7349, 9.9912) (-3.7368, 10.0005) (-3.7384, 10.0084) (-3.7403, 10.0178) (-3.7423, 10.0272) (-3.744, 10.0354) (-3.7461, 10.0449) (-3.7482, 10.0545) (-3.7501, 10.0628) (-3.7523, 10.0725) (-3.7546, 10.0823) (-3.7566, 10.0908) (-3.759, 10.1007) (-3.7615, 10.1106) (-3.7636, 10.1192) (-3.7662, 10.1293) (-3.7688, 10.1394) (-3.7711, 10.1481) (-3.7738, 10.1583) (-3.7765, 10.1686) (-3.779, 10.1774) (-3.7819, 10.1878) (-3.7848, 10.1982) (-3.7874, 10.2072) (-3.7904, 10.2177) (-3.7936, 10.2283) (-3.7963, 10.2374) (-3.7995, 10.2481) (-3.8028, 10.2588) (-3.8057, 10.268) (-3.8091, 10.2789) (-3.8125, 10.2897) (-3.8155, 10.2991) (-3.8191, 10.31) (-3.8228, 10.321) (-3.8259, 10.3305) (-3.8297, 10.3415) (-3.8335, 10.3527) (-3.8368, 10.3622) (-3.8408, 10.3734) (-3.8448, 10.3847) (-3.8483, 10.3943) (-3.8524, 10.4057) (-3.8566, 10.417) (-3.8602, 10.4268) (-3.8645, 10.4382) (-3.8689, 10.4497) (-3.8727, 10.4596) (-3.8772, 10.4711) (-3.8817, 10.4827) (-3.8857, 10.4927) (-3.8897, 10.5027) (-3.8958, 10.5177) (-3.9013, 10.5311) (-3.9069, 10.5446) (-3.9125, 10.5581) (-3.9198, 10.5751) (-3.9249, 10.587) (-3.9301, 10.5989) (-3.9354, 10.6109) (-3.9423, 10.6263) (-3.9477, 10.6384) (-3.9532, 10.6504) (-3.9595, 10.6643) (-3.966, 10.6781) (-3.9709, 10.6886) (-3.9758, 10.699) (-3.9808, 10.7095) (-3.985, 10.7182) (-3.9893, 10.727) (-3.9936, 10.7358) (-3.9979, 10.7446) (-4.0022, 10.7533) (-4.0066, 10.7622) (-4.011, 10.771) (-4.0154, 10.7798) (-4.0199, 10.7887) (-4.0244, 10.7975) (-4.029, 10.8064) (-4.0336, 10.8153) (-4.0382, 10.8242) (-4.0428, 10.8331) (-4.0475, 10.842) (-4.0523, 10.851) (-4.057, 10.8599) (-4.0618, 10.8689) (-4.0667, 10.8778) (-4.0715, 10.8868) (-4.0764, 10.8958) (-4.0814, 10.9048) (-4.0864, 10.9138) (-4.0914, 10.9228) (-4.0964, 10.9318) (-4.1035, 10.9445) (-4.1097, 10.9554) (-4.1149, 10.9644) (-4.119, 10.9717) (-4.1222, 10.9771) knots 0 0 0 0 0 0 0.004167 0.008333 0.0125 0.016667 0.020833 0.025 0.029167 0.033333 0.0375 0.041667 0.045833 0.05 0.054167 0.058333 0.0625 0.066667 0.070833 0.075 0.079167 0.083333 0.0875 0.091667 0.095833 0.1 0.104167 0.108333 0.1125 0.116667 0.120833 0.125 0.129167 0.1375 0.141667 0.145833 0.154167 0.158333 0.1625 0.170833 0.175 0.179167 0.1875 0.191667 0.195833 0.204167 0.208333 0.2125 0.220833 0.225 0.229167 0.2375 0.241667 0.245833 0.254167 0.258333 0.2625 0.270833 0.275 0.279167 0.2875 0.291667 0.295833 0.304167 0.308333 0.3125 0.320833 0.325 0.329167 0.3375 0.341667 0.345833 0.354167 0.358333 0.3625 0.370833 0.375 0.379167 0.3875 0.391667 0.395833 0.404167 0.408333 0.4125 0.420833 0.425 0.429167 0.4375 0.441667 0.445833 0.454167 0.458333 0.4625 0.470833 0.475 0.479167 0.4875 0.491667 0.495833 0.504167 0.508333 0.5125 0.520833 0.525 0.529167 0.5375 0.541667 0.545833 0.554167 0.558333 0.5625 0.570833 0.575 0.579167 0.5875 0.591667 0.595833 0.604167 0.608333 0.6125 0.620833 0.625 0.629167 0.6375 0.641667 0.645833 0.654167 0.658333 0.6625 0.670833 0.675 0.679167 0.6875 0.691667 0.695833 0.704167 0.708333 0.7125 0.720833 0.725 0.729167 0.7375 0.741667 0.745833 0.754167 0.758333 0.7625 0.770833 0.775 0.779167 0.783333 0.8 0.804167 0.808333 0.8125 0.825 0.829167 0.833333 0.8375 0.85 0.854167 0.858333 0.866667 0.870833 0.875 0.879167 0.883333 0.8875 0.891667 0.895833 0.9 0.904167 0.908333 0.9125 0.916667 0.920833 0.925 0.929167 0.933333 0.9375 0.941667 0.945833 0.95 0.954167 0.958333 0.9625 0.966667 0.970833 0.975 0.979167 0.983333 0.9875 1 1 1 1 1 1
  line L28 (-5.343, 9.6404) -> (-5.2725, 8.755)
  line L29 (-5.3431, 9.641) -> (-5.343, 9.6404)
  arc A14 (-4.1222, 10.9771) -> (-4.7415, 11.0183) centre (-4.8955, 4.02) ccw
  arc A15 (-5.2725, 8.755) -> (-6.3511, 8.5415) centre (-4.8955, 4.02) ccw
  spline S14 degree 5 poles (-4.7415, 11.0183) (-4.7454, 11.0133) (-4.7505, 11.0067) (-4.7568, 10.9984) (-4.7643, 10.9884) (-4.7731, 10.9768) (-4.7793, 10.9685) (-4.7854, 10.9602) (-4.7916, 10.952) (-4.7976, 10.9437) (-4.8037, 10.9355) (-4.8097, 10.9272) (-4.8157, 10.9189) (-4.8216, 10.9107) (-4.8275, 10.9025) (-4.8334, 10.8942) (-4.8392, 10.886) (-4.845, 10.8778) (-4.8508, 10.8696) (-4.8565, 10.8614) (-4.8622, 10.8532) (-4.8678, 10.845) (-4.8735, 10.8368) (-4.879, 10.8287) (-4.8846, 10.8205) (-4.8901, 10.8123) (-4.8955, 10.8042) (-4.901, 10.7961) (-4.9064, 10.7879) (-4.9117, 10.7798) (-4.9181, 10.7701) (-4.9244, 10.7604) (-4.9307, 10.7507) (-4.938, 10.7394) (-4.9451, 10.7281) (-4.9513, 10.7184) (-4.9573, 10.7088) (-4.9633, 10.6992) (-4.9692, 10.6896) (-4.9751, 10.68) (-4.981, 10.6704) (-4.9877, 10.6592) (-4.9944, 10.6481) (-5.0001, 10.6386) (-5.0066, 10.6275) (-5.0131, 10.6165) (-5.0186, 10.607) (-5.0249, 10.596) (-5.0312, 10.585) (-5.0365, 10.5756) (-5.0427, 10.5647) (-5.0488, 10.5538) (-5.0539, 10.5445) (-5.0607, 10.5321) (-5.0674, 10.5198) (-5.0732, 10.509) (-5.0789, 10.4982) (-5.0862, 10.4845) (-5.0917, 10.4738) (-5.0972, 10.4632) (-5.1027, 10.4526) (-5.1095, 10.439) (-5.1148, 10.4285) (-5.12, 10.418) (-5.1259, 10.406) (-5.1316, 10.3942) (-5.1359, 10.3853) (-5.1408, 10.3749) (-5.1457, 10.3646) (-5.1498, 10.3558) (-5.1545, 10.3456) (-5.1592, 10.3354) (-5.1631, 10.3268) (-5.1676, 10.3167) (-5.1721, 10.3066) (-5.1759, 10.298) (-5.1802, 10.288) (-5.1845, 10.2781) (-5.1881, 10.2696) (-5.1923, 10.2598) (-5.1964, 10.25) (-5.1998, 10.2416) (-5.2038, 10.2319) (-5.2077, 10.2222) (-5.211, 10.214) (-5.2148, 10.2044) (-5.2185, 10.1949) (-5.2217, 10.1867) (-5.2253, 10.1773) (-5.2288, 10.1679) (-5.2318, 10.1599) (-5.2353, 10.1506) (-5.2386, 10.1414) (-5.2415, 10.1335) (-5.2447, 10.1244) (-5.2479, 10.1153) (-5.2506, 10.1076) (-5.2537, 10.0986) (-5.2567, 10.0897) (-5.2592, 10.0821) (-5.2621, 10.0734) (-5.265, 10.0646) (-5.2673, 10.0572) (-5.2701, 10.0486) (-5.2728, 10.04) (-5.275, 10.0327) (-5.2776, 10.0243) (-5.2801, 10.0159) (-5.2822, 10.0088) (-5.2846, 10.0005) (-5.2869, 9.9923) (-5.2889, 9.9853) (-5.2911, 9.9773) (-5.2933, 9.9693) (-5.2951, 9.9625) (-5.2972, 9.9546) (-5.2992, 9.9468) (-5.3009, 9.9402) (-5.3029, 9.9326) (-5.3047, 9.925) (-5.3063, 9.9185) (-5.3081, 9.9111) (-5.3098, 9.9037) (-5.3112, 9.8975) (-5.3129, 9.8903) (-5.3145, 9.8831) (-5.3158, 9.8771) (-5.3173, 9.8701) (-5.3187, 9.8632) (-5.3199, 9.8573) (-5.3212, 9.8505) (-5.3225, 9.8439) (-5.3236, 9.8382) (-5.3248, 9.8317) (-5.326, 9.8253) (-5.327, 9.8198) (-5.328, 9.8136) (-5.3291, 9.8074) (-5.3299, 9.8022) (-5.3309, 9.7962) (-5.3318, 9.7903) (-5.3326, 9.7853) (-5.3334, 9.7796) (-5.3342, 9.7739) (-5.3349, 9.7692) (-5.3356, 9.7637) (-5.3363, 9.7584) (-5.3368, 9.7538) (-5.3374, 9.7487) (-5.338, 9.7436) (-5.3385, 9.7394) (-5.339, 9.7345) (-5.3395, 9.7297) (-5.3399, 9.7257) (-5.3403, 9.7218) (-5.3407, 9.7167) (-5.3411, 9.7123) (-5.3414, 9.7075) (-5.3418, 9.7028) (-5.3421, 9.6983) (-5.3423, 9.695) (-5.3425, 9.6918) (-5.3426, 9.6892) (-5.3427, 9.6866) (-5.3429, 9.6841) (-5.343, 9.6817) (-5.3431, 9.6793) (-5.3431, 9.677) (-5.3432, 9.6748) (-5.3433, 9.6726) (-5.3433, 9.6705) (-5.3434, 9.6685) (-5.3434, 9.6665) (-5.3434, 9.6646) (-5.3435, 9.6628) (-5.3435, 9.661) (-5.3435, 9.6593) (-5.3435, 9.6576) (-5.3435, 9.6561) (-5.3435, 9.6546) (-5.3435, 9.6531) (-5.3434, 9.6518) (-5.3434, 9.6505) (-5.3434, 9.6493) (-5.3434, 9.6481) (-5.3433, 9.6471) (-5.3433, 9.6461) (-5.3433, 9.6452) (-5.3432, 9.6443) (-5.3432, 9.6436) (-5.3432, 9.6429) (-5.3431, 9.6422) (-5.3431, 9.6417) (-5.3431, 9.6413) (-5.3431, 9.6411) (-5.3431, 9.641) knots -1 -1 -1 -1 -1 -1 -0.9875 -0.983333 -0.979167 -0.975 -0.970833 -0.966667 -0.9625 -0.958333 -0.954167 -0.95 -0.945833 -0.941667 -0.9375 -0.933333 -0.929167 -0.925 -0.920833 -0.916667 -0.9125 -0.908333 -0.904167 -0.9 -0.895833 -0.891667 -0.8875 -0.883333 -0.879167 -0.875 -0.870833 -0.8625 -0.858333 -0.854167 -0.845833 -0.841667 -0.8375 -0.833333 -0.829167 -0.820833 -0.816667 -0.8125 -0.804167 -0.8 -0.795833 -0.7875 -0.783333 -0.779167 -0.770833 -0.766667 -0.7625 -0.754167 -0.75 -0.745833 -0.733333 -0.729167 -0.725 -0.720833 -0.708333 -0.704167 -0.7 -0.695833 -0.683333 -0.679167 -0.675 -0.666667 -0.6625 -0.658333 -0.65 -0.645833 -0.641667 -0.633333 -0.629167 -0.625 -0.616667 -0.6125 -0.608333 -0.6 -0.595833 -0.591667 -0.583333 -0.579167 -0.575 -0.566667 -0.5625 -0.558333 -0.55 -0.545833 -0.541667 -0.533333 -0.529167 -0.525 -0.516667 -0.5125 -0.508333 -0.5 -0.495833 -0.491667 -0.483333 -0.479167 -0.475 -0.466667 -0.4625 -0.458333 -0.45 -0.445833 -0.441667 -0.433333 -0.429167 -0.425 -0.416667 -0.4125 -0.408333 -0.4 -0.395833 -0.391667 -0.383333 -0.379167 -0.375 -0.366667 -0.3625 -0.358333 -0.35 -0.345833 -0.341667 -0.333333 -0.329167 -0.325 -0.316667 -0.3125 -0.308333 -0.3 -0.295833 -0.291667 -0.283333 -0.279167 -0.275 -0.266667 -0.2625 -0.258333 -0.25 -0.245833 -0.241667 -0.233333 -0.229167 -0.225 -0.216667 -0.2125 -0.208333 -0.2 -0.195833 -0.191667 -0.183333 -0.179167 -0.175 -0.170833 -0.158333 -0.154167 -0.145833 -0.141667 -0.1375 -0.133333 -0.129167 -0.125 -0.120833 -0.116667 -0.1125 -0.108333 -0.104167 -0.1 -0.095833 -0.091667 -0.0875 -0.083333 -0.079167 -0.075 -0.070833 -0.066667 -0.0625 -0.058333 -0.054167 -0.05 -0.045833 -0.041667 -0.0375 -0.033333 -0.029167 -0.025 -0.020833 -0.016667 -0.0125 -0.008333 0 0 0 0 0 0
  line L30 (-6.3511, 8.5415) -> (-6.6232, 9.3869)
  line L31 (-6.6232, 9.3869) -> (-6.6234, 9.3875)
  line L32 (-8.0932, 8.6636) -> (-7.5895, 7.9321)
  spline S15 degree 5 poles (-6.6234, 9.3875) (-6.6235, 9.3876) (-6.6235, 9.3877) (-6.6236, 9.3879) (-6.6237, 9.3882) (-6.6239, 9.3887) (-6.6241, 9.3893) (-6.6243, 9.39) (-6.6246, 9.3907) (-6.6248, 9.3915) (-6.6252, 9.3923) (-6.6255, 9.3932) (-6.6259, 9.3942) (-6.6263, 9.3953) (-6.6267, 9.3964) (-6.6272, 9.3976) (-6.6277, 9.3989) (-6.6282, 9.4002) (-6.6288, 9.4016) (-6.6294, 9.4031) (-6.63, 9.4046) (-6.6307, 9.4061) (-6.6314, 9.4078) (-6.6321, 9.4095) (-6.6328, 9.4112) (-6.6336, 9.413) (-6.6344, 9.4149) (-6.6353, 9.4168) (-6.6362, 9.4188) (-6.6371, 9.4209) (-6.638, 9.423) (-6.639, 9.4251) (-6.6403, 9.4278) (-6.6415, 9.4305) (-6.6429, 9.4333) (-6.6445, 9.4366) (-6.6462, 9.4401) (-6.6477, 9.4432) (-6.6495, 9.4468) (-6.6514, 9.4505) (-6.653, 9.4538) (-6.655, 9.4577) (-6.6571, 9.4617) (-6.659, 9.4652) (-6.6612, 9.4694) (-6.6635, 9.4736) (-6.6655, 9.4773) (-6.6679, 9.4817) (-6.6704, 9.4862) (-6.6726, 9.4901) (-6.6752, 9.4948) (-6.6779, 9.4995) (-6.6803, 9.5036) (-6.6831, 9.5084) (-6.686, 9.5134) (-6.6886, 9.5176) (-6.6916, 9.5227) (-6.6947, 9.5278) (-6.6975, 9.5323) (-6.7007, 9.5376) (-6.704, 9.5429) (-6.707, 9.5475) (-6.7104, 9.553) (-6.714, 9.5585) (-6.7171, 9.5632) (-6.7208, 9.5689) (-6.7245, 9.5746) (-6.7278, 9.5795) (-6.7317, 9.5853) (-6.7357, 9.5912) (-6.7392, 9.5962) (-6.7433, 9.6022) (-6.7475, 9.6082) (-6.7512, 9.6134) (-6.7555, 9.6195) (-6.76, 9.6257) (-6.7638, 9.631) (-6.7684, 9.6373) (-6.773, 9.6436) (-6.7771, 9.649) (-6.7818, 9.6554) (-6.7867, 9.6619) (-6.7909, 9.6674) (-6.796, 9.674) (-6.801, 9.6805) (-6.8055, 9.6862) (-6.8107, 9.6928) (-6.816, 9.6995) (-6.8206, 9.7053) (-6.8261, 9.7121) (-6.8316, 9.7189) (-6.8364, 9.7247) (-6.8421, 9.7316) (-6.8479, 9.7385) (-6.8528, 9.7444) (-6.8587, 9.7514) (-6.8647, 9.7584) (-6.8699, 9.7644) (-6.876, 9.7715) (-6.8822, 9.7786) (-6.8876, 9.7847) (-6.894, 9.7919) (-6.9004, 9.799) (-6.906, 9.8052) (-6.9125, 9.8124) (-6.9192, 9.8197) (-6.925, 9.8259) (-6.9318, 9.8332) (-6.9386, 9.8406) (-6.9446, 9.8469) (-6.9516, 9.8543) (-6.9587, 9.8616) (-6.9648, 9.868) (-6.9721, 9.8754) (-6.9794, 9.8829) (-6.9857, 9.8893) (-6.9932, 9.8968) (-7.0008, 9.9043) (-7.0073, 9.9108) (-7.015, 9.9183) (-7.0227, 9.9259) (-7.0295, 9.9323) (-7.0374, 9.9399) (-7.0454, 9.9475) (-7.0523, 9.9541) (-7.0604, 9.9617) (-7.0686, 9.9693) (-7.0757, 9.9759) (-7.0841, 9.9835) (-7.0925, 9.9912) (-7.0998, 9.9978) (-7.1083, 10.0055) (-7.117, 10.0132) (-7.1245, 10.0198) (-7.1333, 10.0275) (-7.1421, 10.0352) (-7.1498, 10.0418) (-7.1588, 10.0496) (-7.1679, 10.0573) (-7.1757, 10.064) (-7.185, 10.0717) (-7.1943, 10.0795) (-7.2023, 10.0861) (-7.2118, 10.0939) (-7.2213, 10.1016) (-7.2295, 10.1083) (-7.2392, 10.116) (-7.2489, 10.1238) (-7.2573, 10.1304) (-7.2658, 10.1371) (-7.2786, 10.1471) (-7.29, 10.1559) (-7.3016, 10.1648) (-7.3133, 10.1736) (-7.328, 10.1847) (-7.3384, 10.1925) (-7.3489, 10.2002) (-7.3595, 10.2079) (-7.3747, 10.219) (-7.3869, 10.2278) (-7.3993, 10.2366) (-7.4118, 10.2454) (-7.4243, 10.2542) (-7.4322, 10.2596) (-7.4402, 10.2651) (-7.4481, 10.2706) (-7.4562, 10.2761) (-7.4642, 10.2815) (-7.4723, 10.287) (-7.4804, 10.2924) (-7.4886, 10.2979) (-7.4968, 10.3033) (-7.505, 10.3088) (-7.5133, 10.3142) (-7.5216, 10.3196) (-7.5299, 10.325) (-7.5383, 10.3305) (-7.5467, 10.3359) (-7.5552, 10.3413) (-7.5636, 10.3466) (-7.5722, 10.352) (-7.5807, 10.3574) (-7.5893, 10.3628) (-7.598, 10.3681) (-7.6066, 10.3735) (-7.6153, 10.3788) (-7.6241, 10.3841) (-7.6329, 10.3895) (-7.6417, 10.3948) (-7.6505, 10.4001) (-7.6594, 10.4054) (-7.6719, 10.4128) (-7.6827, 10.4191) (-7.6917, 10.4244) (-7.6989, 10.4286) (-7.7044, 10.4317) knots 0 0 0 0 0 0 0.004167 0.008333 0.0125 0.016667 0.020833 0.025 0.029167 0.033333 0.0375 0.041667 0.045833 0.05 0.054167 0.058333 0.0625 0.066667 0.070833 0.075 0.079167 0.083333 0.0875 0.091667 0.095833 0.1 0.104167 0.108333 0.1125 0.116667 0.120833 0.125 0.129167 0.1375 0.141667 0.145833 0.154167 0.158333 0.1625 0.170833 0.175 0.179167 0.1875 0.191667 0.195833 0.204167 0.208333 0.2125 0.220833 0.225 0.229167 0.2375 0.241667 0.245833 0.254167 0.258333 0.2625 0.270833 0.275 0.279167 0.2875 0.291667 0.295833 0.304167 0.308333 0.3125 0.320833 0.325 0.329167 0.3375 0.341667 0.345833 0.354167 0.358333 0.3625 0.370833 0.375 0.379167 0.3875 0.391667 0.395833 0.404167 0.408333 0.4125 0.420833 0.425 0.429167 0.4375 0.441667 0.445833 0.454167 0.458333 0.4625 0.470833 0.475 0.479167 0.4875 0.491667 0.495833 0.504167 0.508333 0.5125 0.520833 0.525 0.529167 0.5375 0.541667 0.545833 0.554167 0.558333 0.5625 0.570833 0.575 0.579167 0.5875 0.591667 0.595833 0.604167 0.608333 0.6125 0.620833 0.625 0.629167 0.6375 0.641667 0.645833 0.654167 0.658333 0.6625 0.670833 0.675 0.679167 0.6875 0.691667 0.695833 0.704167 0.708333 0.7125 0.720833 0.725 0.729167 0.7375 0.741667 0.745833 0.754167 0.758333 0.7625 0.770833 0.775 0.779167 0.783333 0.8 0.804167 0.808333 0.8125 0.825 0.829167 0.833333 0.8375 0.854167 0.858333 0.8625 0.866667 0.870833 0.875 0.879167 0.883333 0.8875 0.891667 0.895833 0.9 0.904167 0.908333 0.9125 0.916667 0.920833 0.925 0.929167 0.933333 0.9375 0.941667 0.945833 0.95 0.954167 0.958333 0.9625 0.966667 0.970833 0.975 0.979167 0.983333 0.9875 1 1 1 1 1 1
  spline S16 degree 5 poles (-8.2613, 10.1577) (-8.2621, 10.1514) (-8.2632, 10.1431) (-8.2646, 10.1328) (-8.2661, 10.1204) (-8.2679, 10.106) (-8.2691, 10.0957) (-8.2703, 10.0855) (-8.2715, 10.0752) (-8.2726, 10.065) (-8.2737, 10.0549) (-8.2748, 10.0447) (-8.2759, 10.0346) (-8.2769, 10.0245) (-8.2779, 10.0144) (-8.2788, 10.0043) (-8.2798, 9.9943) (-8.2807, 9.9843) (-8.2816, 9.9743) (-8.2824, 9.9643) (-8.2833, 9.9544) (-8.2841, 9.9445) (-8.2848, 9.9346) (-8.2856, 9.9247) (-8.2863, 9.9149) (-8.287, 9.9051) (-8.2876, 9.8953) (-8.2883, 9.8855) (-8.2889, 9.8758) (-8.2895, 9.8661) (-8.2901, 9.8544) (-8.2907, 9.8429) (-8.2913, 9.8313) (-8.292, 9.8179) (-8.2925, 9.8045) (-8.293, 9.7931) (-8.2934, 9.7818) (-8.2938, 9.7704) (-8.2941, 9.7591) (-8.2945, 9.7479) (-8.2947, 9.7367) (-8.295, 9.7236) (-8.2952, 9.7107) (-8.2954, 9.6996) (-8.2955, 9.6867) (-8.2956, 9.6739) (-8.2956, 9.663) (-8.2956, 9.6503) (-8.2956, 9.6376) (-8.2955, 9.6268) (-8.2953, 9.6125) (-8.2951, 9.5983) (-8.2949, 9.5859) (-8.2946, 9.5735) (-8.2941, 9.5578) (-8.2937, 9.5455) (-8.2933, 9.5334) (-8.2928, 9.5213) (-8.2921, 9.5059) (-8.2916, 9.494) (-8.2909, 9.4821) (-8.2903, 9.4703) (-8.2894, 9.4552) (-8.2886, 9.4436) (-8.2878, 9.432) (-8.2868, 9.4188) (-8.2858, 9.4058) (-8.285, 9.396) (-8.2841, 9.3847) (-8.2831, 9.3734) (-8.2822, 9.3639) (-8.2811, 9.3527) (-8.28, 9.3417) (-8.279, 9.3323) (-8.2778, 9.3214) (-8.2766, 9.3105) (-8.2756, 9.3013) (-8.2743, 9.2906) (-8.273, 9.2799) (-8.2718, 9.2709) (-8.2705, 9.2604) (-8.2691, 9.2499) (-8.2678, 9.241) (-8.2664, 9.2307) (-8.2649, 9.2205) (-8.2636, 9.2118) (-8.262, 9.2017) (-8.2605, 9.1917) (-8.2591, 9.1832) (-8.2574, 9.1734) (-8.2558, 9.1636) (-8.2543, 9.1552) (-8.2526, 9.1456) (-8.2509, 9.136) (-8.2494, 9.1279) (-8.2476, 9.1185) (-8.2458, 9.1092) (-8.2442, 9.1012) (-8.2424, 9.092) (-8.2405, 9.0829) (-8.2389, 9.0752) (-8.237, 9.0662) (-8.235, 9.0574) (-8.2333, 9.0498) (-8.2314, 9.0411) (-8.2294, 9.0325) (-8.2277, 9.0252) (-8.2256, 9.0167) (-8.2236, 9.0083) (-8.2218, 9.0012) (-8.2198, 8.9929) (-8.2177, 8.9848) (-8.2159, 8.9779) (-8.2138, 8.9699) (-8.2116, 8.962) (-8.2098, 8.9553) (-8.2077, 8.9476) (-8.2055, 8.94) (-8.2037, 8.9335) (-8.2015, 8.9261) (-8.1993, 8.9187) (-8.1974, 8.9124) (-8.1952, 8.9052) (-8.193, 8.8981) (-8.1912, 8.8921) (-8.1889, 8.8852) (-8.1867, 8.8783) (-8.1848, 8.8725) (-8.1826, 8.8659) (-8.1804, 8.8593) (-8.1785, 8.8538) (-8.1763, 8.8474) (-8.1741, 8.8411) (-8.1722, 8.8358) (-8.17, 8.8297) (-8.1678, 8.8237) (-8.166, 8.8186) (-8.1638, 8.8128) (-8.1616, 8.8071) (-8.1597, 8.8022) (-8.1576, 8.7967) (-8.1554, 8.7913) (-8.1536, 8.7867) (-8.1515, 8.7815) (-8.1494, 8.7763) (-8.1476, 8.772) (-8.1455, 8.7671) (-8.1435, 8.7622) (-8.1417, 8.7582) (-8.1397, 8.7536) (-8.1377, 8.749) (-8.136, 8.7452) (-8.134, 8.7409) (-8.1321, 8.7367) (-8.1305, 8.7332) (-8.1286, 8.7292) (-8.1268, 8.7253) (-8.1252, 8.722) (-8.1234, 8.7183) (-8.1217, 8.7147) (-8.1202, 8.7118) (-8.1187, 8.7089) (-8.1173, 8.7061) (-8.1161, 8.7038) (-8.115, 8.7016) (-8.1139, 8.6994) (-8.1128, 8.6974) (-8.1117, 8.6953) (-8.1106, 8.6933) (-8.1096, 8.6914) (-8.1086, 8.6896) (-8.1076, 8.6878) (-8.1067, 8.6861) (-8.1057, 8.6844) (-8.1048, 8.6828) (-8.104, 8.6812) (-8.1031, 8.6798) (-8.1023, 8.6783) (-8.1015, 8.677) (-8.1007, 8.6757) (-8.1, 8.6745) (-8.0993, 8.6733) (-8.0987, 8.6722) (-8.098, 8.6712) (-8.0974, 8.6702) (-8.0969, 8.6693) (-8.0964, 8.6684) (-8.0959, 8.6677) (-8.0954, 8.667) (-8.095, 8.6663) (-8.0946, 8.6657) (-8.0943, 8.6651) (-8.094, 8.6647) (-8.0938, 8.6644) (-8.0937, 8.6642) (-8.0936, 8.6641) knots -1 -1 -1 -1 -1 -1 -0.9875 -0.983333 -0.979167 -0.975 -0.970833 -0.966667 -0.9625 -0.958333 -0.954167 -0.95 -0.945833 -0.941667 -0.9375 -0.933333 -0.929167 -0.925 -0.920833 -0.916667 -0.9125 -0.908333 -0.904167 -0.9 -0.895833 -0.891667 -0.8875 -0.883333 -0.879167 -0.875 -0.870833 -0.8625 -0.858333 -0.854167 -0.845833 -0.841667 -0.8375 -0.833333 -0.829167 -0.820833 -0.816667 -0.8125 -0.804167 -0.8 -0.795833 -0.7875 -0.783333 -0.779167 -0.770833 -0.766667 -0.7625 -0.75 -0.745833 -0.741667 -0.7375 -0.725 -0.720833 -0.716667 -0.7125 -0.7 -0.695833 -0.691667 -0.6875 -0.675 -0.670833 -0.666667 -0.658333 -0.654167 -0.65 -0.641667 -0.6375 -0.633333 -0.625 -0.620833 -0.616667 -0.608333 -0.604167 -0.6 -0.591667 -0.5875 -0.583333 -0.575 -0.570833 -0.566667 -0.558333 -0.554167 -0.55 -0.541667 -0.5375 -0.533333 -0.525 -0.520833 -0.516667 -0.508333 -0.504167 -0.5 -0.491667 -0.4875 -0.483333 -0.475 -0.470833 -0.466667 -0.458333 -0.454167 -0.45 -0.441667 -0.4375 -0.433333 -0.425 -0.420833 -0.416667 -0.408333 -0.404167 -0.4 -0.391667 -0.3875 -0.383333 -0.375 -0.370833 -0.366667 -0.358333 -0.354167 -0.35 -0.341667 -0.3375 -0.333333 -0.325 -0.320833 -0.316667 -0.308333 -0.304167 -0.3 -0.291667 -0.2875 -0.283333 -0.275 -0.270833 -0.266667 -0.258333 -0.254167 -0.25 -0.241667 -0.2375 -0.233333 -0.225 -0.220833 -0.216667 -0.208333 -0.204167 -0.2 -0.191667 -0.1875 -0.183333 -0.175 -0.170833 -0.166667 -0.158333 -0.154167 -0.15 -0.141667 -0.1375 -0.133333 -0.129167 -0.125 -0.120833 -0.116667 -0.1125 -0.108333 -0.104167 -0.1 -0.095833 -0.091667 -0.0875 -0.083333 -0.079167 -0.075 -0.070833 -0.066667 -0.0625 -0.058333 -0.054167 -0.05 -0.045833 -0.041667 -0.0375 -0.033333 -0.029167 -0.025 -0.020833 -0.016667 -0.0125 -0.008333 0 0 0 0 0 0
  arc A16 (-7.7044, 10.4317) -> (-8.2613, 10.1577) centre (-4.8955, 4.02) ccw
  line L33 (-8.0936, 8.6641) -> (-8.0932, 8.6636)
  arc A17 (-9.1847, 6.061) -> (-9.539, 5.0202) centre (-4.8955, 4.02) ccw
  line L34 (-9.9866, 6.4426) -> (-9.1847, 6.061)
  line L35 (-9.9872, 6.4429) -> (-9.9866, 6.4426)